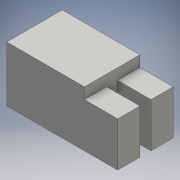
# Autodesk Inventor part: connectiontest1
Saved by Autodesk Inventor 2016 (Build 200138000, 138)
## iProperties
Created: 2015-11-19
Part Number: connectiontest1
Material: Generic
Document SubType Name: Modeling
Designer: hesaon
Density: 1 g/cm^3
Appearance: Default
Author: hesaon
Autodesk Inventor part; units mm, degrees
ref_plane "YZ Plane" through (0, 0, 0) normal (1, 0, 0) x (0, 1, 0)
ref_plane "XZ Plane" through (0, 0, 0) normal (0, 1, 0) x (-1, 0, 0)
ref_plane "XY Plane" through (0, 0, 0) normal (0, 0, 1) x (1, 0, 0)
sketch "Sketch1" plane through (0, 0, 0) normal (0, 0, 1) x (1, 0, 0)
  line L0 (0, 0) -> (-40, 0)
  line L1 (-40, 0) -> (-40, 20)
  line L2 (-40, 20) -> (0, 20)
  line L3 (0, 20) -> (0, 0)
  dimension "d0" = 40
  dimension "d1" = 20
  constraints: 8 end point, 2 parallel, 1 horizontal, 1 perpendicular
  measures "d0" distance of L1.end L2.end
  measures "d1" distance of L0.end L1.end
extrude "Extrusion1" add sketch "Sketch1" along normal blind 20
sketch "Sketch2" plane through (-40, 20, 0) normal (0, 1, 0) x (1, 0, 0)
  line L0 (0, -20) -> (40, -20) projected
  line L1 (40, -20) -> (40, -16)
  line L2 (40, 0) -> (40, -20) projected
  line L3 (28, -20) -> (28, -16)
  line L4 (28, -16) -> (40, -16)
  dimension "d4" = 4
  dimension "d5" = 12
  constraints: 6 end point, 2 point on line, 1 perpendicular, 1 vertical
  measures "d4" distance of L0.end L1.end
  measures "d5" distance of L1.end L3.end
extrude "Extrusion2" cut sketch "Sketch2" against normal through all
sketch "Sketch3" plane through (0, 0, 0) normal (1, 0, 0) x (0, 0, -1)
  line L0 (-16, 20) -> (-16, 0) projected
  line L1 (-16, 12) -> (0, 12)
  line L2 (0, 20) -> (0, 0) projected
  line L3 (0, 8) -> (-16, 8)
  dimension "d8" = 8
  dimension "d9" = 8
  constraints: 4 end point, 4 point on line, 1 horizontal, 1 parallel
  measures "d8" distance of L2.start L1.end
  measures "d9" distance of L2.end L3.start
extrude "Extrusion3" cut sketch "Sketch3" against normal blind 12
body "Solid1"
